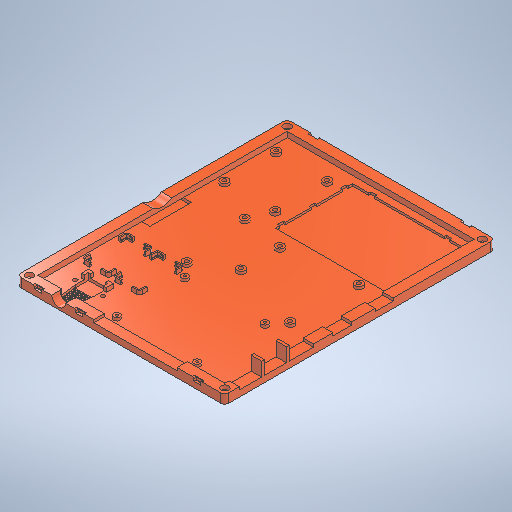
# Autodesk Inventor part: Electronic Base - Final
Saved by Autodesk Inventor 2025.2 (Build 292293000, 293)
## iProperties
Created: 2025-03-21
Part Number: Electronic Base - Final
Material: Generic
Document SubType Name: Modeling
Designer: mnguyen6
Density: 1 g/cm^3
Appearance: Default
Author: mnguyen6
Autodesk Inventor part; units mm, degrees
ref_plane "YZ Plane" through (0, 0, 0) normal (1, 0, 0) x (0, 1, 0)
ref_plane "XZ Plane" through (0, 0, 0) normal (0, 1, 0) x (-1, 0, 0)
ref_plane "XY Plane" through (0, 0, 0) normal (0, 0, 1) x (1, 0, 0)
sketch "Sketch1" plane through (0, 0, 0) normal (0, 1, 0) x (-1, 0, 0)
  line L0 (0, 0) -> (-135, 0)
  line L1 (-135, 0) -> (-135, 180)
  line L2 (-135, 180) -> (0, 180)
  line L3 (0, 180) -> (0, 0)
  line L4 (7.5, -7.5) -> (-142.5, -7.5)
  line L5 (-142.5, -7.5) -> (-142.5, 187.5)
  line L6 (-142.5, 187.5) -> (7.5, 187.5)
  line L7 (7.5, 187.5) -> (7.5, -7.5)
  line L8 (-31.4, 118) -> (-133, 118) construction
  line L9 (-133, 118) -> (-133, 64.66) construction
  line L10 (-133, 64.66) -> (-31.4, 64.66) construction
  line L11 (-31.4, 64.66) -> (-31.4, 118) construction
  circle A0 centre (-117.76, 115.46) radius 1.4
  circle A1 centre (-119.03, 67.2) radius 1.4
  circle A2 centre (-66.96, 100.22) radius 1.4
  circle A3 centre (-66.96, 72.28) radius 1.4
  circle A4 centre (-42.83, 115.46) radius 1.4
  circle A5 centre (-36.48, 67.2) radius 1.4
  circle A6 centre (-117.76, 115.46) radius 2.9
  circle A7 centre (-119.03, 67.2) radius 2.9
  circle A8 centre (-66.96, 72.28) radius 2.9
  circle A9 centre (-66.96, 100.22) radius 2.9
  circle A10 centre (-42.83, 115.46) radius 2.9
  circle A11 centre (-36.48, 67.2) radius 2.9
  line L12 (-134.5, 60.3514) -> (-52.82, 60.3514) construction
  line L13 (-52.82, 60.3514) -> (-52.82, 5.6014) construction
  line L14 (-52.82, 5.6014) -> (-134.5, 5.6014) construction
  line L15 (-134.5, 5.6014) -> (-134.5, 60.3514) construction
  line L16 (-52.32, 5.1014) -> (-52.32, 60.8514)
  line L17 (-52.32, 60.8514) -> (-135, 60.8514)
  line L18 (-135, 60.8514) -> (-135, 5.1014)
  line L19 (-135, 5.1014) -> (-52.32, 5.1014)
  line L20 (-52.32, 34.9764) -> (-50.82, 34.9764)
  line L21 (-50.82, 34.9764) -> (-50.82, 30.9764)
  line L22 (-50.82, 30.9764) -> (-52.32, 30.9764)
  line L23 (-52.32, 30.9764) -> (-52.32, 34.9764)
  line L24 (-52.32, 12.2764) -> (-50.82, 12.2764)
  line L25 (-50.82, 12.2764) -> (-50.82, 8.2764)
  line L26 (-50.82, 8.2764) -> (-52.32, 8.2764)
  line L27 (-52.32, 57.6764) -> (-50.82, 57.6764)
  line L28 (-50.82, 57.6764) -> (-50.82, 53.6764)
  line L29 (-50.82, 53.6764) -> (-52.32, 53.6764)
  line L30 (-118.6, 5.1014) -> (-122.6, 5.1014)
  line L31 (-122.6, 5.1014) -> (-122.6, 3.6014)
  line L32 (-122.6, 3.6014) -> (-118.6, 3.6014)
  line L33 (-118.6, 3.6014) -> (-118.6, 5.1014)
  line L34 (-68.07, 5.1014) -> (-64.07, 5.1014)
  line L35 (-64.07, 5.1014) -> (-64.07, 3.6014)
  line L36 (-64.07, 3.6014) -> (-68.07, 3.6014)
  line L37 (-68.07, 3.6014) -> (-68.07, 5.1014)
  line L38 (-48, 178) -> (-133, 178) construction
  line L39 (-133, 178) -> (-133, 122) construction
  line L40 (-133, 122) -> (-48, 122) construction
  line L41 (-48, 122) -> (-48, 178) construction
  circle A12 centre (-51.5, 174.5) radius 0.9
  circle A13 centre (-51.5, 125.5) radius 0.9
  circle A14 centre (-109.5, 174.5) radius 0.9
  circle A15 centre (-109.5, 125.5) radius 0.9
  circle A16 centre (-51.5, 174.5) radius 2.4
  circle A17 centre (-51.5, 125.5) radius 2.4
  circle A18 centre (-109.5, 174.5) radius 2.4
  circle A19 centre (-109.5, 125.5) radius 2.4
  line L42 (-5.087, 151.3381) -> (-22.387, 151.3381)
  line L43 (-22.387, 151.3381) -> (-22.387, 121.0381)
  line L44 (-22.387, 121.0381) -> (-5.087, 121.0381)
  line L45 (-5.087, 121.0381) -> (-5.087, 151.3381)
  line L46 (-2.73, 54.1134) -> (-45.73, 54.1134) construction
  line L47 (-45.73, 54.1134) -> (-45.73, 11.1134) construction
  line L48 (-45.73, 11.1134) -> (-2.73, 11.1134) construction
  line L49 (-2.73, 11.1134) -> (-2.73, 54.1134) construction
  line L50 (-27.387, 151.3381) -> (-44.687, 151.3381)
  line L51 (-44.687, 151.3381) -> (-44.687, 121.0381)
  line L52 (-44.687, 121.0381) -> (-27.387, 121.0381)
  line L53 (-27.387, 121.0381) -> (-27.387, 151.3381)
  circle A20 centre (-6.05, 13.9844) radius 1.4
  circle A21 centre (-6.05, 13.9844) radius 2.9
  circle A22 centre (-42.787, 13.9844) radius 2.9
  circle A23 centre (-42.787, 13.9844) radius 1.4
  circle A24 centre (-6.05, 51.3574) radius 1.4
  circle A25 centre (-6.05, 51.3574) radius 2.9
  circle A26 centre (-42.787, 51.3574) radius 2.9
  circle A27 centre (-42.787, 51.3574) radius 1.4
  line L54 (-22.5, 178.166) -> (-22.5, 163.2053) construction
  line L55 (-27.75, 181.5) -> (-29.5, 168.5)
  line L56 (-15.5, 168.5) -> (-17.25, 181.5)
  line L57 (-17.25, 181.5) -> (-27.75, 181.5)
  line L58 (-15.5, 168.5) -> (-15.5, 159)
  line L59 (-15.5, 159) -> (-29.5, 159)
  line L60 (-29.5, 159) -> (-29.5, 168.5)
  line L61 (-27.9654, 179.9) -> (-17.0346, 179.9)
  line L62 (-28.0731, 179.1) -> (-16.9269, 179.1)
  line L63 (-28.2346, 177.9) -> (-16.7654, 177.9)
  line L64 (-28.3423, 177.1) -> (-16.6577, 177.1)
  line L65 (-28.5038, 175.9) -> (-16.4962, 175.9)
  line L66 (-16.3885, 175.1) -> (-28.6115, 175.1)
  line L67 (-28.7731, 173.9) -> (-16.2269, 173.9)
  line L68 (-16.1192, 173.1) -> (-28.8808, 173.1)
  line L69 (-29.0423, 171.9) -> (-15.9577, 171.9)
  line L70 (-29.15, 171.1) -> (-15.85, 171.1)
  line L71 (-29.3115, 169.9) -> (-15.6885, 169.9)
  line L72 (-15.5808, 169.1) -> (-29.4192, 169.1)
  line L73 (-17.25, 159) -> (-27.75, 159)
  line L74 (-27.75, 159) -> (-27.75, 154.5)
  line L75 (-27.75, 154.5) -> (-17.25, 154.5)
  line L76 (-17.25, 154.5) -> (-17.25, 159)
  line L77 (-15.5, 162) -> (-13.5, 162)
  line L78 (-13.5, 162) -> (-13.5, 157)
  line L79 (-13.5, 157) -> (-17, 157)
  line L80 (-17, 157) -> (-17, 159)
  line L81 (-29.5, 162) -> (-31.5, 162)
  line L82 (-31.5, 162) -> (-31.5, 157)
  line L83 (-31.5, 157) -> (-28, 157)
  line L84 (-28, 157) -> (-28, 159)
  line L85 (-26.387, 152.3381) -> (-45.687, 152.3381)
  line L86 (-45.687, 152.3381) -> (-45.687, 120.0381)
  line L87 (-45.687, 120.0381) -> (-26.387, 120.0381)
  line L88 (-26.387, 120.0381) -> (-26.387, 152.3381)
  line L89 (-27.887, 150.8381) -> (-44.187, 150.8381)
  line L90 (-44.187, 150.8381) -> (-44.187, 121.5381)
  line L91 (-44.187, 121.5381) -> (-27.887, 121.5381)
  line L92 (-27.887, 121.5381) -> (-27.887, 150.8381)
  line L93 (-4.087, 152.3381) -> (-23.387, 152.3381)
  line L94 (-23.387, 152.3381) -> (-23.387, 120.0381)
  line L95 (-23.387, 120.0381) -> (-4.087, 120.0381)
  line L96 (-4.087, 120.0381) -> (-4.087, 152.3381)
  line L97 (-5.587, 150.8381) -> (-21.887, 150.8381)
  line L98 (-21.887, 150.8381) -> (-21.887, 121.5381)
  line L99 (-21.887, 121.5381) -> (-5.587, 121.5381)
  line L100 (-5.587, 121.5381) -> (-5.587, 150.8381)
  line L101 (-31.887, 152.3381) -> (-31.887, 150.8381)
  line L102 (-31.887, 120.0381) -> (-31.887, 121.5381)
  line L103 (-9.587, 152.3381) -> (-9.587, 150.8381)
  line L104 (-9.587, 121.5381) -> (-9.587, 120.0381)
  line L105 (-40.187, 152.3381) -> (-40.187, 150.8381)
  line L106 (-17.887, 121.5381) -> (-17.887, 120.0381)
  line L107 (-40.187, 121.5381) -> (-40.187, 120.0381)
  line L108 (-17.887, 152.3381) -> (-17.887, 150.8381)
  line L109 (-26.387, 146.8381) -> (-27.887, 146.8381)
  line L110 (-44.187, 146.8381) -> (-45.687, 146.8381)
  line L111 (-26.387, 125.5381) -> (-27.887, 125.5381)
  line L112 (-44.187, 125.5381) -> (-45.687, 125.5381)
  line L113 (-4.087, 146.8381) -> (-5.587, 146.8381)
  line L114 (-21.887, 146.8381) -> (-23.387, 146.8381)
  line L115 (-4.087, 125.5381) -> (-5.587, 125.5381)
  line L116 (-21.887, 125.5381) -> (-23.387, 125.5381)
  circle A28 centre (-12.5, 165.5) radius 1.5
  circle A29 centre (-32.5, 165.5) radius 1.5
  point P0 (-50.82, 32.9764)
  point P1 (-52.32, 32.9764)
  point P2 (-50.82, 10.2764)
  point P3 (-50.82, 55.6764)
  point P4 (-22.5, 154.5)
  point P5 (-22.5, 159)
  point P6 (-27.9519, 180)
  point P7 (-17.0481, 180)
  point P8 (-135, 5.1014)
  point P9 (-64.07, 5.1014)
  point P10 (-52.32, 8.2764)
  point P11 (-52.32, 12.2764)
  point P12 (-52.32, 30.9764)
  point P13 (-52.32, 57.6764)
  point P14 (-135, 60.8514)
  point P15 (-27.387, 125.5381)
  point P16 (-31.887, 121.0381)
  point P17 (-44.687, 125.5381)
  point P18 (-40.187, 121.0381)
  point P19 (-27.387, 146.8381)
  point P20 (-31.887, 151.3381)
  point P21 (-44.687, 146.8381)
  point P22 (-40.187, 151.3381)
  point P23 (-5.087, 125.5381)
  point P24 (-9.587, 121.0381)
  point P25 (-22.387, 125.5381)
  point P26 (-17.887, 121.0381)
  point P27 (-5.087, 146.8381)
  point P28 (-9.587, 151.3381)
  point P29 (-22.387, 146.8381)
  point P30 (-17.887, 151.3381)
  point P31 (-27.75, 159)
  point P32 (-28, 159)
  point P33 (-29.5, 162)
  dimension "d0" = 7.5
  dimension "d1" = 53.34
  dimension "d2" = 101.6
  dimension "d3" = 15.24
  dimension "d4" = 13.97
  dimension "d5" = 2.54
  dimension "d6" = 50.8
  dimension "d7" = 17.78
  dimension "d9" = 66.04
  dimension "d10" = 90.17
  dimension "d11" = 96.52
  dimension "d12" = 45.72
  dimension "d13" = 2.8
  dimension "d15" = 54.75
  dimension "d16" = 81.68
  dimension "d17" = 0.5
  dimension "d18" = 4
  dimension "d19" = 1.5
  dimension "d22" = 22.7
  dimension "d27" = 11.9
  dimension "d28" = 54.53
  dimension "d29" = 2
  dimension "d31" = 56
  dimension "d32" = 85
  dimension "d33" = 3.5
  dimension "d34" = 3.5
  dimension "d35" = 1.8
  dimension "d37" = 52.5
  dimension "d38" = 61.5
  dimension "d39" = 1.5
  dimension "d40" = 2
  dimension "d44" = 43
  dimension "d46" = 17.3
  dimension "d49" = 30.3
  dimension "d50" = 2.871
  dimension "d51" = 3.32
  dimension "d52" = 2.8
  dimension "d54" = 1.5
  dimension "d55" = 1.5
  dimension "d56" = 40.244
  dimension "d57" = 40.057
  dimension "d59" = 10.5
  dimension "d62" = 6
  dimension "d63" = 14
  dimension "d64" = 30
  dimension "d65" = 1.6
  dimension "d66" = 0.8
  dimension "d67" = 1.2
  dimension "d68" = 0.8
  dimension "d69" = 1.2
  dimension "d70" = 0.8
  dimension "d71" = 1.2
  dimension "d72" = 0.8
  dimension "d73" = 1.2
  dimension "d74" = 0.8
  dimension "d75" = 1.2
  dimension "d76" = 0.8
  dimension "d77" = 9.5
  dimension "d78" = 13
  dimension "d79" = 10.5
  dimension "d80" = 4.5
  dimension "d81" = 3
  dimension "d82" = 2
  dimension "d83" = 2
  constraints: 230 end point, 41 parallel, 38 point on line, 30 centre point, 27 perpendicular, 23 horizontal, 22 equal radius, 13 coincident, 12 collinear, 10 vertical, 8 equal length, 8 horizontal alignment, 6 symmetric about line, 6 vertical alignment, 4 midpoint, 65 other
  measures "d0" distance between parallel lines of L3 L7
  measures "d1" distance of L8.end L9.end
  measures "d2" distance of L9.end L10.end
  measures "d3" distance from line of L9 A0.centre
  measures "d4" distance from line of L9 A1.centre
  measures "d5" distance from line of L8 A0.centre
  measures "d6" distance from line of A1.centre L8
  measures "d7" distance from line of A2.centre L8
  measures "d9" distance from line of L9 A2.centre
  measures "d10" horizontal distance of L9.end A4.centre
  measures "d11" horizontal distance of L9.end A5.centre
  measures "d12" vertical distance of L8.end A3.centre
  measures "d13" diameter of A0
  measures "d15" distance of L14.end L12.start
  measures "d16" distance of L13.end L14.end
  measures "d17" distance between parallel lines of L13 L16
  measures "d18" distance of L20.end L21.end
  measures "d19" distance of L21.end L22.end
  measures "d22" distance of L20.start L24.start
  measures "d27" distance between parallel lines of L15 L31
  measures "d28" distance of L31.end L36.end
  measures "d29" distance between parallel lines of L1 L9
  measures "d31" distance of L38.end L39.end
  measures "d32" distance of L38.start L38.end
  measures "d33" distance from line of L38 A12.centre
  measures "d34" distance from line of L41 A12.centre
  measures "d35" diameter of A12
  measures "d37" vertical distance of L38.start A13.centre
  measures "d38" distance from line of L41 A14.centre
  measures "d39" radial gap between concentric circles of A12 A16
  measures "d40" distance between parallel lines of L2 L38
  measures "d44" distance of L46.end L47.end
  measures "d46" distance of L50.start L50.end
  measures "d49" distance of L50.end L51.end
  measures "d50" distance from line of L48 A20.centre
  measures "d51" horizontal distance of L48.end A20.centre
  measures "d52" diameter of A20
  measures "d54" radial gap between concentric circles of A21 A20
  measures "d55" radial gap between concentric circles of A6 A0
  measures "d56" distance from line of A24.centre L48
  measures "d57" horizontal distance of A22.centre L48.end
  measures "d59" distance of L57.start L57.end
  measures "d62" distance between parallel lines of L6 L57
  measures "d63" distance of L58.end L59.end
  measures "d64" distance between parallel lines of L7 L54
  measures "d65" distance between parallel lines of L57 L61
  measures "d66" distance between parallel lines of L61 L62
  measures "d67" distance between parallel lines of L63 L62
  measures "d68" distance between parallel lines of L64 L63
  measures "d69" distance between parallel lines of L64 L65
  measures "d70" distance between parallel lines of L65 L66
  measures "d71" distance between parallel lines of L66 L67
  measures "d72" distance between parallel lines of L67 L68
  measures "d73" distance between parallel lines of L68 L69
  measures "d74" distance between parallel lines of L69 L70
  measures "d75" distance between parallel lines of L70 L71
  measures "d76" distance between parallel lines of L71 L72
  measures "d77" distance of L58.end L58.start
  measures "d78" vertical distance of L57.start L58.start
  measures "d79" distance of L74.end L75.end
  measures "d80" distance of L73.end L74.end
  measures "d81" distance of L58.end L77.start
  measures "d82" distance of L77.start L77.end
  measures "d83" distance of L79.end L80.end
extrude "Base" add sketch "Sketch1" against normal blind 2.5 contours L0 L1 L19 L31 L32 L33 L37 L36 L35 L16 L26 L25 L24 L22 L21 L20 L29 L28 L27 L17 L2 L55 L60 L81 L82 L83 L84 L59 L74 L75 L76 L80 L79 L78 L77 L58 L56 L3 | L1 L17 L16 L19 | L56 L61 L55 L2 | L2 L55 L57 L56 | L19 L33 L32 L31 | L56 L62 L55 L61 | L56 L63 L55 L62 | L27 L28 L29 L16 | L19 L35 L36 L37 | L56 L64 L55 L63 | L56 L65 L55 L64 | L20 L21 L22 L16 | L56 L66 L55 L65 | L16 L24 L25 L26 | L56 L67 L55 L66 | L56 L68 L55 L67 | L56 L69 L55 L68 | L56 L70 L55 L69 | L56 L71 L55 L70 | L56 L72 L55 L71 | L56 L58 L59 L60 L55 L72 | L77 L78 L79 L80 L59 L58 | L60 L59 L84 L83 L82 L81 | L76 L75 L74 L59 | L4 L5 L6 L7 | A0 | A1 | A2 | A3 | A4 | A5 | A6 | A7 | A8 | A9 | A10 | A11 | A12 | A13 | A14 | A15 | A16 | A17 | A18 | A19 | L45 L113 L100 L97 L103 L42 | L42 L103 L93 L96 L113 L45 | L103 L97 L108 L42 | L42 L108 L93 L103 | L113 L96 L115 L45 | L45 L115 L100 L113 | L108 L97 L98 L114 L43 L42 | L42 L43 L114 L94 L93 L108 | L97 L100 L99 L98 | L115 L96 L95 L104 L44 L45 | L45 L44 L104 L99 L100 L115 | L114 L98 L116 L43 | L43 L116 L94 L114 | L104 L95 L106 L44 | L44 L106 L99 L104 | L116 L98 L99 L106 L44 L43 | L43 L44 L106 L95 L94 L116 | L53 L109 L92 L89 L101 L50 | L50 L101 L85 L88 L109 L53 | L101 L89 L105 L50 | L50 L105 L85 L101 | L109 L88 L111 L53 | L53 L111 L92 L109 | L105 L89 L90 L110 L51 L50 | L50 L51 L110 L86 L85 L105 | L89 L92 L91 L90 | L111 L88 L87 L102 L52 L53 | L53 L52 L102 L91 L92 L111 | L110 L90 L112 L51 | L51 L112 L86 L110 | L102 L87 L107 L52 | L52 L107 L91 L102 | L112 L90 L91 L107 L52 L51 | L51 L52 L107 L87 L86 L112 | A20 | A21 | A22 | A23 | A24 | A25 | A26 | A27 | A28 | A29
extrude "Wall" add sketch "Sketch1" along normal blind 4 contours L4 L5 L6 L7
extrude "Breadboard slot" cut sketch "Sketch1" against normal blind 1.5 contours L1 L17 L16 L19 | L19 L33 L32 L31 | L27 L28 L29 L16 | L19 L35 L36 L37 | L20 L21 L22 L16 | L16 L24 L25 L26
extrude "Mounting hole wall" add sketch "Sketch1" along normal blind 2 contours A6 | A7 | A8 | A9 | A10 | A11 | A16 | A17 | A18 | A19 | A21 | A22 | A25 | A26
extrude "Deeper mounting holes" cut sketch "Sketch1" against normal blind 1 contours A0 | A1 | A2 | A3 | A4 | A5 | A12 | A13 | A14 | A15 | A20 | A23 | A24 | A27
extrude "Extrusion14" cut sketch "Sketch1" against normal through all contours A28 | A29
extrude "MT3608 base" add sketch "Sketch1" along normal blind 1 contours L45 L113 L100 L97 L103 L42 | L108 L97 L98 L114 L43 L42 | L45 L44 L104 L99 L100 L115 | L116 L98 L99 L106 L44 L43 | L53 L109 L92 L89 L101 L50 | L105 L89 L90 L110 L51 L50 | L53 L52 L102 L91 L92 L111 | L112 L90 L91 L107 L52 L51
extrude "MT3608 wall" add sketch "Sketch1" along normal blind 3 contours L42 L103 L93 L96 L113 L45 | L42 L43 L114 L94 L93 L108 | L115 L96 L95 L104 L44 L45 | L43 L44 L106 L95 L94 L116 | L50 L101 L85 L88 L109 L53 | L50 L51 L110 L86 L85 L105 | L111 L88 L87 L102 L52 L53 | L51 L52 L107 L87 L86 L112
sketch "Sketch2" plane through (31.887, 0, 150.8381) normal (1, 0, 0) x (0, 0, -1)
  line L0 (-0.5, 1) -> (-0.5, 3) projected
  line L1 (-0.5, 3) -> (0, 2.5)
  line L2 (0, 2.5) -> (-0.5, 2)
  line L3 (0, 2.5) -> (-0.5, 2.5) construction
  point P0 (150.8381, 0)
  dimension "d108" = 1
  dimension "d109" = 45
  constraints: 6 end point, 1 midpoint, 1 perpendicular, 1 point on line, 1 other
  measures "d108" distance of L0.start L2.end
  measures "d109" angle of L0 L2
extrude "MT3608 snap" add sketch "Sketch2" against normal blind 2
ref_plane "Work Plane1" through (31.887, 0, 136.1881) normal (0, 0, -1) x (-1, 0, 0)
ref_plane "Work Plane2" through (36.037, 0, 152.3381) normal (-1, 0, 0) x (0, 0, 1)
fillet "Fillet1" radius 0.3 1 edges at (30.887, 2.5, 150.8381)
mirror "Mirror1" about plane through (31.887, 0, 136.1881) normal (0, 0, -1) of "MT3608 snap", "Fillet1"
mirror "Mirror2" about plane through (36.037, 0, 152.3381) normal (-1, 0, 0) of "MT3608 snap", "Mirror1", "Fillet1"
ref_plane "Work Plane3" through (24.887, 0, 146.8381) normal (1, 0, 0) x (0, 0, -1)
mirror "Mirror3" about plane through (24.887, 0, 146.8381) normal (1, 0, 0) of "MT3608 snap", "Fillet1", "Mirror1", "Mirror2"
fillet "Fillet2" radius 2 8 edges at (26.387, 1.5, 152.3381) (26.387, 1.5, 120.0381) (4.087, 1.5, 152.3381) (4.087, 1.5, 120.0381) (45.687, 1.5, 152.3381) (45.687, 1.5, 120.0381) (23.387, 1.5, 152.3381) (23.387, 1.5, 120.0381)
extrude "Extrusion9" cut sketch "Sketch1" against normal blind 2 contours L56 L61 L55 L2 | L2 L55 L57 L56 | L56 L62 L55 L61 | L56 L63 L55 L62 | L56 L64 L55 L63 | L56 L65 L55 L64 | L56 L66 L55 L65 | L56 L67 L55 L66 | L56 L68 L55 L67 | L56 L69 L55 L68 | L56 L70 L55 L69 | L56 L71 L55 L70 | L56 L72 L55 L71 | L56 L58 L59 L60 L55 L72
extrude "Extrusion10" add sketch "Sketch1" along normal blind 0.5 from surface at -2 contours L56 L61 L55 L2 | L56 L62 L55 L61 | L56 L64 L55 L63 | L56 L66 L55 L65 | L56 L68 L55 L67 | L56 L70 L55 L69 | L56 L72 L55 L71
extrude "Extrusion11" add sketch "Sketch1" along normal blind 3 contours L77 L78 L79 L80 L59 L58 | L60 L59 L84 L83 L82 L81
sketch "Sketch4" plane through (0, 4, 0) normal (0, 1, 0) x (1, 0, 0)
  line L0 (142.5, -187.5) -> (142.5, 7.5) projected
  line L1 (135, 0) -> (135, -180) projected
  line L2 (48, -178) -> (133, -178) construction
  line L3 (135, -177) -> (142.5, -177)
  line L4 (142.5, -177) -> (142.5, -161)
  line L5 (142.5, -161) -> (135, -161)
  line L6 (135, -161) -> (135, -177)
  line L7 (135, -159) -> (142.5, -159)
  line L8 (142.5, -159) -> (142.5, -143)
  line L9 (142.5, -143) -> (135, -143)
  line L10 (135, -143) -> (135, -159)
  line L11 (135, -141) -> (142.5, -141)
  line L12 (142.5, -141) -> (142.5, -123.5)
  line L13 (142.5, -123.5) -> (135, -123.5)
  line L14 (135, -123.5) -> (135, -141)
  line L15 (31.4, -118) -> (133, -118) construction
  line L16 (135, -109.5) -> (142.5, -109.5)
  line L17 (142.5, -109.5) -> (142.5, -95.86)
  line L18 (142.5, -95.86) -> (135, -95.86)
  line L19 (135, -95.86) -> (135, -109.5)
  line L20 (135, -79) -> (142.5, -79)
  line L21 (142.5, -79) -> (142.5, -66)
  line L22 (142.5, -66) -> (135, -66)
  line L23 (135, -66) -> (135, -79)
  line L24 (-7.5, -187.5) -> (142.5, -187.5) projected
  line L25 (135, -180) -> (27.9519, -180) projected
  line L26 (48, -187.5) -> (108, -187.5)
  line L27 (108, -187.5) -> (108, -180)
  line L28 (108, -180) -> (48, -180)
  line L29 (48, -180) -> (48, -187.5)
  line L30 (133, -178) -> (133, -122) construction
  point P0 (135, -66)
  point P1 (142.5, -109.5)
  point P2 (142.5, -177)
  point P3 (108, -187.5)
  dimension "d125" = 1
  dimension "d127" = 19
  dimension "d129" = 37
  dimension "d131" = 8.5
  dimension "d132" = 13.64
  dimension "d133" = 39
  dimension "d134" = 13
  dimension "d137" = 25
  dimension "d138" = 85
  dimension "d176" = 17
  dimension "d177" = 35
  dimension "d178" = 54.5
  constraints: 48 end point, 12 parallel, 12 point on line, 6 horizontal, 6 perpendicular
  measures "d125" distance from line of L3.end L2
  measures "d127" vertical distance of L2.end L7.end
  measures "d129" vertical distance of L2.end L11.end
  measures "d131" vertical distance of L15.end L16.end
  measures "d132" distance of L16.end L17.end
  measures "d133" vertical distance of L20.end L15.end
  measures "d134" distance of L20.end L21.end
  measures "d137" horizontal distance of L2.end L26.end
  measures "d138" distance from line of L30 L26.start
  measures "d176" distance between parallel lines of L5 L2
  measures "d177" distance between parallel lines of L2 L9
  measures "d178" distance from line of L2.end L13
extrude "Board Ports" cut sketch "Sketch4" against normal blind 2 contours L3 L1 L5 L0 | L24 L29 L25 L27 | L7 L1 L9 L0 | L11 L1 L13 L0 | L16 L1 L18 L0 | L20 L1 L22 L0
extrude "Extrusion22" add sketch "Sketch4" along normal blind 8 contours L5 L1 L7 L0 | L9 L1 L11 L0
sketch "Sketch5" plane through (27.75, 4, 181.5) normal (0, 0, -1) x (-1, 0, 0)
  line L0 (0, 0) -> (10.5, 0) projected
  line L1 (0, -6) -> (10.5, -6) projected
  circle A0 centre (5.25, 0) radius 5
  point P0 (27.75, -4)
  point P1 (5.25, -5)
  point P2 (5.25, -5)
  dimension "d139" = 10
  constraints: 1 centre point, 1 midpoint
  measures "d139" diameter of A0
extrude "DC jack opening" cut sketch "Sketch5" against normal through all
fillet "Fillet3" radius 3 4 edges at (-7.5, 0.75, 187.5) (-7.5, 0.75, -7.5) (142.5, 0.75, 187.5) (142.5, 0.75, -7.5)
ref_plane "Work Plane4" through (122.5, 4, 123.5) normal (1, 0, 0) x (0, 0, -1)
ref_plane "Work Plane5" through (37.5, 4, 123.5) normal (1, 0, 0) x (0, 0, -1)
ref_plane "Work Plane6" through (12.5, 4, 123.5) normal (1, 0, 0) x (0, 0, -1)
ref_plane "Work Plane7" through (7.5, 4, 123.5) normal (1, 0, 0) x (0, 0, -1)
sketch "Sketch6" plane through (142.5, 4, 123.5) normal (1, 0, 0) x (0, 0, -1)
  line L0 (128, -6.5) -> (-61, -6.5) projected
  line L1 (-64, 0) -> (-56.5, 0) projected
  line L2 (-64, 0) -> (-62.5, 0)
  line L3 (-62.5, 0) -> (-62.5, -2.5)
  line L4 (-62.5, -2.5) -> (-64, -2.5)
  line L5 (-64, -2.5) -> (-64, 0)
  line L6 (-62.5, -2.5) -> (-61.5, -1.5)
  line L7 (-61.5, -1.5) -> (-62.5, -0.5)
  line L8 (-61.5, -1.5) -> (-62.5, -1.5) construction
  line L9 (33.5, 7.7447) -> (33.5, -39.6927) construction
  line L10 (131, 0) -> (129.5, 0)
  line L11 (129.5, 0) -> (129.5, -2.5)
  line L12 (129.5, -2.5) -> (131, -2.5)
  line L13 (131, -2.5) -> (131, 0)
  line L14 (129.5, -2.5) -> (128.5, -1.5)
  line L15 (128.5, -1.5) -> (129.5, -0.5)
  line L16 (128.5, -1.5) -> (129.5, -1.5) construction
  point P0 (123.5, -4)
  point P1 (33.5, -6.5)
  point P2 (-62.5, 0)
  dimension "d148" = 1.5
  dimension "d149" = 2.5
  dimension "d150" = 1
  dimension "d151" = 45
  constraints: 30 end point, 7 symmetric about line, 5 point on line, 2 parallel, 2 perpendicular, 1 horizontal, 1 midpoint, 1 vertical, 1 other
  measures "d148" distance of L1.start L2.end
  measures "d149" distance of L4.end L1.start
  measures "d150" distance of L6.end L8.end
  measures "d151" angle of L3 L6
extrude "Snap fit point 1" cut sketch "Sketch6" along normal mid plane 5 from surface at -20 contours L1 L3 L4 L5 | L7 L6 L3
extrude "Snap fit point 2" cut sketch "Sketch6" along normal mid plane 5 from surface at -105 contours L1 L3 L4 L5 | L7 L6 L3
extrude "Snap fit point 3" cut sketch "Sketch6" along normal mid plane 5 from surface at -135 contours L1 L3 L4 L5 | L7 L6 L3
extrude "Snap fit point 4" cut sketch "Sketch6" along normal mid plane 5 from surface at -130 contours L13 L12 L11 L10 | L11 L14 L15
extrude "Snap fit point 5" cut sketch "Sketch6" along normal mid plane 5 from surface at -20 contours L13 L12 L11 L10 | L11 L14 L15
sketch "Sketch7" plane through (0, 0, 0) normal (1, 0, 0) x (0, 0, -1)
  line L0 (0, 0) -> (-180, 0) projected
  circle A0 centre (-90, 13) radius 11.25
  line L1 (0, 0) -> (0, 4) projected
  dimension "d169" = 22.5
  dimension "d170" = 13
  dimension "d182" = 90
  constraints: 1 centre point
  measures "d169" diameter of A0
  measures "d170" distance from line of L0 A0.centre
  measures "d182" distance from line of L1 A0.centre
extrude "Cable opening" cut sketch "Sketch7" against normal through all
fillet "Fillet4" radius 1 5 edges at (122.5, 2.5, 185) (37.5, 2.5, 185) (7.5, 2.5, 185) (122.5, 2.5, -5) (12.5, 2.5, -5)
sketch "Sketch11" plane through (0, 0, 0) normal (0, 1, 0) x (1, 0, 0)
  line L0 (-14.5812, -90) -> (16.6397, -90) construction
  line L1 (0, -83.25) -> (0, -96.75) projected
  line L2 (-2.0532, -105) -> (5.9468, -105)
  line L3 (5.9468, -105) -> (5.9468, -75)
  line L4 (5.9468, -75) -> (-2.0532, -75)
  line L5 (-2.0532, -75) -> (-2.0532, -105)
  point P0 (0, -90)
  point P1 (5.9468, -90)
  dimension "d184" = 30
  dimension "d185" = 8
  constraints: 10 end point, 2 horizontal, 2 midpoint, 2 parallel, 2 point on line, 1 perpendicular
  measures "d184" distance of L2.end L3.end
  measures "d185" distance of L3.end L4.end
extrude "Slot for cable gland nut" cut sketch "Sketch11" against normal blind 2
fillet "Fillet5" radius 1 10 edges at (10, 4, -6.75) (15, 4, -6.75) (120, 4, -6.75) (125, 4, -6.75) (125, 4, 186.75) (120, 4, 186.75) (40, 4, 186.75) (35, 4, 186.75) (10, 4, 186.75) (5, 4, 186.75)
sketch "Sketch12" plane through (0, -2.5, 0) normal (0, -1, 0) x (1, 0, 0)
  line L0 (139.5, 187.5) -> (-4.5, 187.5) projected
  line L1 (-7.5, 184.5) -> (-7.5, -4.5) projected
  line L2 (-0.1, 181.3257) -> (-3, 179.6514)
  line L3 (-3, 179.6514) -> (-5.9, 181.3257)
  line L4 (-5.9, 181.3257) -> (-5.9, 184.6743)
  line L5 (-5.9, 184.6743) -> (-3, 186.3486)
  line L6 (-3, 186.3486) -> (-0.1, 184.6743)
  line L7 (-0.1, 184.6743) -> (-0.1, 181.3257)
  circle A0 centre (-3, 183) radius 2.75
  circle A1 centre (-3, 183) radius 1.6
  point P0 (0, 0)
  dimension "d189" = 5.8
  dimension "d190" = 4.5
  dimension "d191" = 4.5
  dimension "d192" = 5.5
  dimension "d195" = 3.2
  constraints: 12 end point, 2 centre point, 2 coincident, 1 vertical, 13 other
  measures "d189" distance between parallel lines of L2 L5
  measures "d190" distance from line of L0 point (-3, 183)
  measures "d191" distance from line of L1 point (-3, 183)
  measures "d192" diameter of A0
  measures "d195" diameter of A1
extrude "Extrusion24" cut sketch "Sketch12" against normal blind 1 contours L2 L3 L4 L5 L6 L7 | A0 | A1
extrude "Extrusion25" cut sketch "Sketch12" against normal through all contours A1
extrude "Extrusion26" cut sketch "Sketch12" along normal blind 3 from surface at -6.5 contours A0
ref_plane "Work Plane8" through (48, 2, 90) normal (0, 0, 1) x (1, 0, 0)
ref_plane "Work Plane9" through (67.5, -2.5, -4.5) normal (-1, 0, 0) x (0, 0, 1)
mirror "Mirror4" about plane through (67.5, -2.5, -4.5) normal (-1, 0, 0) of "Extrusion25", "Extrusion24", "Extrusion26"
mirror "Mirror5" about plane through (48, 2, 90) normal (0, 0, 1) of "Extrusion26", "Extrusion25", "Extrusion24", "Mirror4"
equation "\"d1\" = MEGA_width"
equation "\"d2\" = MEGA_length"
equation "\"d3\" = MEGA_hole1_y"
equation "\"d4\" = MEGA_hole2_y"
equation "\"d5\" = MEGA_hole1_x"
equation "\"d6\" = MEGA_hole2_x"
equation "\"d7\" = MEGA_hole3_x"
equation "\"d9\" = MEGA_hole3_y"
equation "\"d10\" = MEGA_hole5_y"
equation "\"d11\" = MEGA_hole6_y"
equation "\"d12\" = MEGA_hole4_x"
equation "\"d29\" = base_border"
equation "\"d31\" = Pi_width"
equation "\"d32\" = Pi_length"
equation "\"d33\" = Pi_hole1_x"
equation "\"d34\" = Pi_hole1_y"
equation "\"d37\" = Pi_hole2_x"
equation "\"d38\" = Pi_hole3_y"
equation "\"d40\" = base_border"
equation "\"d44\" = L298N_width"
equation "\"MEGA_width\" = 53.34"
equation "\"MEGA_length\" = 101.6"
equation "\"MEGA_hole1_y\" = 15.24"
equation "\"MEGA_hole1_x\" = 2.54"
equation "\"MEGA_hole2_x\" = 50.8"
equation "\"MEGA_hole2_y\" = 13.97"
equation "\"MEGA_hole3_x\" = 17.78"
equation "\"MEGA_hole3_y\" = 66.04"
equation "\"MEGA_hole4_x\" = 45.72"
equation "\"MEGA_hole5_y\" = 90.17"
equation "\"MEGA_hole6_y\" = 96.52"
equation "\"Pi_width\" = 56"
equation "\"Pi_length\" = 85"
equation "\"Pi_hole1_x\" = 3.5"
equation "\"Pi_hole1_y\" = 3.5"
equation "\"Pi_hole2_x\" = 52.5"
equation "\"Pi_hole3_y\" = 61.5"
equation "\"base_border\" = 2"
equation "\"MT3608_width\" = 17"
equation "\"L298N_width\" = 43"
equation "\"d48\" = 17"
equation "\"mount_hole_wall\" = 1.5"
body "Solid1"
